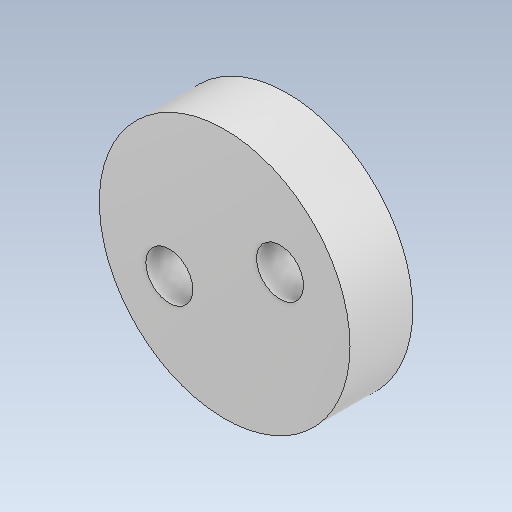
# Autodesk Inventor part: 原動節-従動節つなぎ
Saved by Autodesk Inventor 2020.4 (Build 244396000, 396)
## iProperties
Created: 2021-05-01
Part Number: 原動節-従動節つなぎ
Material: アルミニウム 2014-T4
Document SubType Name: Modeling
Designer: happy
Density: 2.8 g/cm^3
Appearance: サテン
Mass: 2.09356 g
Surface Area: 6.5031 cm^2
Volume: 0.747699 cm^3
Author: happy
Autodesk Inventor part; units mm, degrees
ref_plane "YZ Plane" through (0, 0, 0) normal (1, 0, 0) x (0, 1, 0)
ref_plane "XZ Plane" through (0, 0, 0) normal (0, 1, 0) x (-1, 0, 0)
ref_plane "XY Plane" through (0, 0, 0) normal (0, 0, 1) x (1, 0, 0)
sketch "スケッチ1" plane through (0, 0, 0) normal (0, 0, 1) x (1, 0, 0)
  circle A0 centre (156.4674, 58.1236) radius 3
  line L0 (156.4674, 58.1236) -> (163.5326, 61.8764) construction
  circle A1 centre (156.4674, 58.1236) radius 4 construction
  circle A2 centre (160, 60) radius 4 construction
  circle A3 centre (163.5326, 61.8764) radius 3
  circle A4 centre (160, 60) radius 8
  circle A5 centre (163.5326, 61.8764) radius 4 construction
  line L1 (161.8764, 56.4674) -> (158.1236, 63.5326) construction
  circle A6 centre (156.4674, 58.1236) radius 1.5
  circle A7 centre (163.5326, 61.8764) radius 1.5
  point P0 (0, 0)
  point P1 (160, 60)
  point P2 (160, 60)
  point P3 (160, 60)
  dimension "d0" = 16
  dimension "d1" = 8
  dimension "d2" = 6
  dimension "d3" = 6
  dimension "d4" = 3
  dimension "d5" = 3
  constraints: 8 centre point, 5 coincident, 5 point on circle, 4 end point, 4 midpoint, 2 tangent, 1 equal radius, 1 point on line, 2 other
  measures "d0" diameter of A4
  measures "d1" diameter of A1
  measures "d2" diameter of A0
  measures "d3" diameter of A3
  measures "d4" diameter of A6
  measures "d5" diameter of A7
extrude "押し出し1" add sketch "スケッチ1" along normal blind 4 contours A0 | A3 | A4
